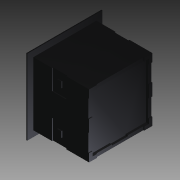
# Autodesk Inventor part: UB216KKW015C-NR
Saved by Autodesk Inventor 2015 SP1 (Build 190203100, 203)
## iProperties
Category: Electrical
Company: Autodesk Inc.
Created: 2014-12-16
Part Number: UB216KKW015C-NR
Catalog Web Link: http://www.nkkswitches.com/
Description: PC and Snap-in Mount Non-Illuminated Pushbuttons_ni_body-Non-Illuminated Pushbuttons - Series UB2
Vendor: NKK Switches
Document SubType Name: Modeling
Designer: Autodesk Inc.
Manufacturer: NKKSWITCHES
Mass: 2.73712 g
Surface Area: 20.1935 cm^2
Volume: 2.73712 cm^3
Density: 1 g/cm^3
Material: Generic
Appearance: PSOLRGB-192-192-192
Title: UB21KK015C-5Cni_body
Author: Autodesk Inc.
Comments: Non-Illuminated Pushbuttons - Series UB2
Autodesk Inventor part; units mm, degrees
sketch "Sketch_11" plane through (1.016, 0, 0) normal (1, 0, 0) x (0, 0, -1)
  line L0 (-9.4996, 9.4996) -> (-9.4996, -9.4996)
  line L1 (-9.4996, -9.4996) -> (9.4996, -9.4996)
  line L2 (9.4996, -9.4996) -> (9.4996, 9.4996)
  line L3 (9.4996, 9.4996) -> (-9.4996, 9.4996)
  constraints: 8 end point
extrude "Extrusion1" add sketch "Sketch_11" against normal blind 15.494
sketch "Sketch_12" plane through (0, 0, 0) normal (0, 0, 1) x (1, 0, 0)
  line L0 (-20.32, 12.8016) -> (-20.32, -12.8016)
  line L1 (-20.32, -12.8016) -> (1.016, -12.8016)
  line L2 (1.016, -12.8016) -> (1.016, -7.9756)
  line L3 (1.016, -7.9756) -> (-13.081, -7.9756)
  line L4 (-13.081, -7.9756) -> (-13.081, -9.4996)
  line L5 (-13.081, -9.4996) -> (-13.335, -9.4996)
  line L6 (-13.335, -9.4996) -> (-14.478, -8.3566)
  line L7 (-14.478, -8.3566) -> (-14.478, 8.3566)
  line L8 (-14.478, 8.3566) -> (-13.335, 9.4996)
  line L9 (-13.335, 9.4996) -> (-13.081, 9.4996)
  line L10 (-13.081, 9.4996) -> (-13.081, 7.9756)
  line L11 (-13.081, 7.9756) -> (1.016, 7.9756)
  line L12 (1.016, 7.9756) -> (1.016, 12.8016)
  line L13 (1.016, 12.8016) -> (-20.32, 12.8016)
  constraints: 28 end point
extrude "Extrusion2" cut sketch "Sketch_12" along normal mid plane 18.9992
sketch "Sketch_13" plane through (0, 0, 0) normal (0, 1, 0) x (-1, 0, 0)
  line L0 (20.32, -12.8016) -> (20.32, 12.8016)
  line L1 (20.32, 12.8016) -> (-1.016, 12.8016)
  line L2 (-1.016, 12.8016) -> (-1.016, 7.9756)
  line L3 (-1.016, 7.9756) -> (13.081, 7.9756)
  line L4 (13.081, 7.9756) -> (13.081, 9.4996)
  line L5 (13.081, 9.4996) -> (13.335, 9.4996)
  line L6 (13.335, 9.4996) -> (14.478, 8.3566)
  line L7 (14.478, 8.3566) -> (14.478, -8.3566)
  line L8 (14.478, -8.3566) -> (13.335, -9.4996)
  line L9 (13.335, -9.4996) -> (13.081, -9.4996)
  line L10 (13.081, -9.4996) -> (13.081, -7.9756)
  line L11 (13.081, -7.9756) -> (-1.016, -7.9756)
  line L12 (-1.016, -7.9756) -> (-1.016, -12.8016)
  line L13 (-1.016, -12.8016) -> (20.32, -12.8016)
  constraints: 28 end point
extrude "Extrusion3" cut sketch "Sketch_13" along normal mid plane 18.9992
sketch "Sketch_14" plane through (1.016, 0, 0) normal (1, 0, 0) x (0, 0, -1)
  line L0 (-7.112, -7.112) -> (-1.9812, -7.112)
  line L1 (-1.9812, -7.112) -> (-1.9812, -7.366)
  line L2 (-1.9812, -7.366) -> (1.9812, -7.366)
  line L3 (1.9812, -7.366) -> (1.9812, -7.112)
  line L4 (1.9812, -7.112) -> (7.112, -7.112)
  line L5 (7.112, -7.112) -> (7.112, 7.112)
  line L6 (7.112, 7.112) -> (-7.112, 7.112)
  line L7 (-7.112, 7.112) -> (-7.112, -7.112)
  constraints: 16 end point
extrude "Extrusion4" cut sketch "Sketch_14" against normal blind 0.762
sketch "Sketch_15" plane through (0, 0, 7.9756) normal (0, 0, 1) x (1, 0, 0)
  line L0 (0.8128, 5.9436) -> (0.8128, 1.524)
  line L1 (0.8128, 1.524) -> (1.016, 1.524)
  line L2 (1.016, 1.524) -> (1.016, 5.9436)
  line L3 (1.016, 5.9436) -> (0.8128, 5.9436)
  constraints: 8 end point
extrude "Extrusion5" cut sketch "Sketch_15" against normal blind 15.9512
sketch "Sketch_16" plane through (0, 0, 7.9756) normal (0, 0, 1) x (1, 0, 0)
  line L0 (0.8128, -5.9436) -> (1.016, -5.9436)
  line L1 (1.016, -5.9436) -> (1.016, -1.524)
  line L2 (1.016, -1.524) -> (0.8128, -1.524)
  line L3 (0.8128, -1.524) -> (0.8128, -5.9436)
  constraints: 8 end point
extrude "Extrusion6" cut sketch "Sketch_16" against normal blind 15.9512
sketch "Sketch_17" plane through (0, 7.9756, 0) normal (0, 1, 0) x (1, 0, 0)
  line L0 (0.8128, 5.9436) -> (0.8128, -5.9436)
  line L1 (0.8128, -5.9436) -> (1.016, -5.9436)
  line L2 (1.016, -5.9436) -> (1.016, 5.9436)
  line L3 (1.016, 5.9436) -> (0.8128, 5.9436)
  constraints: 8 end point
extrude "Extrusion7" cut sketch "Sketch_17" against normal blind 15.9512
sketch "Sketch_48" plane through (0, 0, 7.9756) normal (0, 0, 1) x (1, 0, 0)
  line L0 (-8.3185, 7.9756) -> (-8.3185, 2.8956)
  line L1 (-8.3185, 2.8956) -> (-4.7625, 2.8956)
  line L2 (-4.7625, 2.8956) -> (-4.7625, 7.9756)
  line L3 (-4.7625, 7.9756) -> (-8.3185, 7.9756)
  line L4 (-7.0485, 6.1976) -> (-7.0485, 4.6736)
  line L5 (-7.0485, 4.6736) -> (-6.0325, 4.6736)
  line L6 (-6.0325, 4.6736) -> (-6.0325, 6.1976)
  line L7 (-6.0325, 6.1976) -> (-7.0485, 6.1976)
  constraints: 16 end point
extrude "Extrusion8" cut sketch "Sketch_48" against normal blind 0.254
sketch "Sketch_50" plane through (0, 0, 7.9756) normal (0, 0, 1) x (1, 0, 0)
  line L0 (-8.3185, -7.9756) -> (-4.7625, -7.9756)
  line L1 (-4.7625, -7.9756) -> (-4.7625, -2.8956)
  line L2 (-4.7625, -2.8956) -> (-8.3185, -2.8956)
  line L3 (-8.3185, -2.8956) -> (-8.3185, -7.9756)
  line L4 (-7.0485, -6.1976) -> (-6.0325, -6.1976)
  line L5 (-6.0325, -6.1976) -> (-6.0325, -4.6736)
  line L6 (-6.0325, -4.6736) -> (-7.0485, -4.6736)
  line L7 (-7.0485, -4.6736) -> (-7.0485, -6.1976)
  constraints: 16 end point
extrude "Extrusion9" cut sketch "Sketch_50" against normal blind 0.254
sketch "Sketch_51" plane through (0, 0, -7.9756) normal (0, 0, 1) x (1, 0, 0)
  line L0 (-8.3185, 7.9756) -> (-8.3185, 2.8956)
  line L1 (-8.3185, 2.8956) -> (-4.7625, 2.8956)
  line L2 (-4.7625, 2.8956) -> (-4.7625, 7.9756)
  line L3 (-4.7625, 7.9756) -> (-8.3185, 7.9756)
  line L4 (-7.0485, 6.1976) -> (-7.0485, 4.6736)
  line L5 (-7.0485, 4.6736) -> (-6.0325, 4.6736)
  line L6 (-6.0325, 4.6736) -> (-6.0325, 6.1976)
  line L7 (-6.0325, 6.1976) -> (-7.0485, 6.1976)
  constraints: 16 end point
extrude "Extrusion10" cut sketch "Sketch_51" along normal blind 0.254
sketch "Sketch_52" plane through (0, 0, -7.9756) normal (0, 0, 1) x (1, 0, 0)
  line L0 (-8.3185, -7.9756) -> (-4.7625, -7.9756)
  line L1 (-4.7625, -7.9756) -> (-4.7625, -2.8956)
  line L2 (-4.7625, -2.8956) -> (-8.3185, -2.8956)
  line L3 (-8.3185, -2.8956) -> (-8.3185, -7.9756)
  line L4 (-7.0485, -6.1976) -> (-6.0325, -6.1976)
  line L5 (-6.0325, -6.1976) -> (-6.0325, -4.6736)
  line L6 (-6.0325, -4.6736) -> (-7.0485, -4.6736)
  line L7 (-7.0485, -4.6736) -> (-7.0485, -6.1976)
  constraints: 16 end point
extrude "Extrusion11" cut sketch "Sketch_52" along normal blind 0.254
sketch "Sketch_21" plane through (-14.478, 0, 0) normal (1, 0, 0) x (0, 0, -1)
  line L0 (-7.5057, -7.5057) -> (7.5057, -7.5057)
  line L1 (7.5057, -7.5057) -> (7.5057, 7.5057)
  line L2 (7.5057, 7.5057) -> (-7.5057, 7.5057)
  line L3 (-7.5057, 7.5057) -> (-7.5057, -7.5057)
  constraints: 8 end point
extrude "Extrusion12" cut sketch "Sketch_21" along normal blind 5.0038
ref_plane "body_to_diffuser_kk23_XY" through (-11.8872, 0, 0) normal (1, 0, 0) x (0, 0, -1)
ref_plane "body_to_diffuser_kk23_YZ" through (-11.8872, 0, 0) normal (0, 0, -1) x (0, 1, 0)
ref_plane "body_to_diffuser_kk23_ZX" through (-11.8872, 0, 0) normal (0, 1, 0) x (1, 0, 0)
ref_plane "body_to_metal_XY" through (-0.508, 0, 0) normal (-1, 0, 0) x (0, 0, -1)
ref_plane "body_to_metal_YZ" through (-0.508, 0, 0) normal (0, 0, -1) x (0, -1, 0)
ref_plane "body_to_metal_ZX" through (-0.508, 0, 0) normal (0, -1, 0) x (-1, 0, 0)
ref_plane "body_to_pole_XY" through (-0.508, 0, 0) normal (-1, 0, 0) x (0, 0, -1)
ref_plane "body_to_pole_YZ" through (-0.508, 0, 0) normal (0, 0, -1) x (0, -1, 0)
ref_plane "body_to_pole_ZX" through (-0.508, 0, 0) normal (0, -1, 0) x (-1, 0, 0)
body "Solid1"
